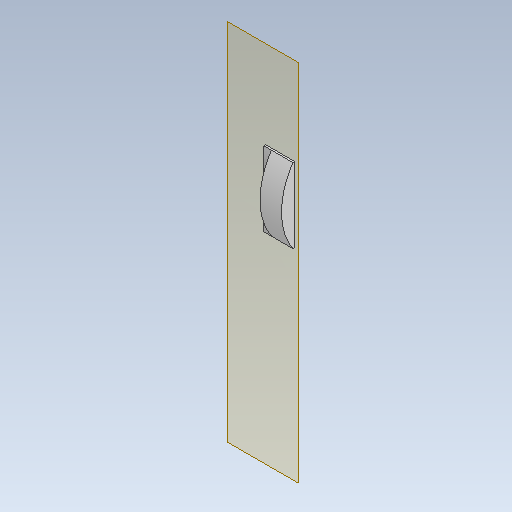
# Autodesk Inventor part: pully cover
Saved by Autodesk Inventor 2020 (Build 240168000, 168)
## iProperties
Created: 2020-03-07
Part Number: pully cover
Material: Generic
Document SubType Name: Modeling
Designer: jackm
Density: 1 g/cm^3
Appearance: Default
Author: jackm
Autodesk Inventor part; units mm, degrees
ref_plane "YZ Plane" through (0, 0, 0) normal (1, 0, 0) x (0, 1, 0)
ref_plane "XZ Plane" through (0, 0, 0) normal (0, 1, 0) x (-1, 0, 0)
ref_plane "XY Plane" through (0, 0, 0) normal (0, 0, 1) x (1, 0, 0)
ref_plane "Work Plane1" through (0, 0, 0) normal (0, 0, 1) x (1, 0, 0)
sketch "Sketch1" plane through (0, 0, 0) normal (0, 0, 1) x (1, 0, 0)
  line L0 (18.4366, 123.794) -> (43.8366, 123.794) construction
  line L1 (18.4366, 32.354) -> (18.4366, 123.794) construction
  line L2 (43.8366, 32.354) -> (18.4366, 32.354) construction
  circle A0 centre (9.9557, 104.744) radius 1.7 construction
  circle A1 centre (9.9557, 51.404) radius 1.7 construction
  line L3 (38.8366, 123.794) -> (18.4366, 123.794)
  line L4 (18.4366, 32.354) -> (38.8366, 32.354)
  circle A2 centre (9.9557, 104.744) radius 1.7
  circle A3 centre (9.9557, 51.404) radius 1.7
  line L5 (4.1111, 104.744) -> (4.1111, 123.794)
  line L6 (4.1111, 104.744) -> (4.1111, 32.354)
  line L7 (38.8366, 225.425) -> (38.8366, -225.425) construction
  line L8 (38.8366, 123.794) -> (38.8366, 32.354)
  line L9 (18.4366, 123.794) -> (18.4366, 32.354)
  line L10 (4.1111, 123.794) -> (4.1111, 128.794)
  line L11 (4.1111, 128.794) -> (43.8366, 128.794)
  line L12 (43.8366, 128.794) -> (43.8366, 32.354)
  line L13 (43.8366, 32.354) -> (43.8366, 27.354)
  line L14 (43.8366, 27.354) -> (4.1111, 27.354)
  line L15 (4.1111, 27.354) -> (4.1111, 32.354)
  point P0 (0, 0)
  dimension "d0" = 3.4
  dimension "d1" = 3.4
  dimension "d2" = 5
  dimension "d3" = 5
  constraints: 24 end point, 6 point on line, 4 perpendicular, 3 collinear, 2 centre point, 2 coincident, 1 parallel, 1 vertical
  measures "d0" diameter of A2
  measures "d1" diameter of A3
  measures "d2" distance of L5.end L10.end
  measures "d3" distance of L2.start L13.end
extrude "Extrusion1" add sketch "Sketch1" along normal blind 2.54
sketch "Sketch2" plane through (38.8366, 32.354, 0) normal (-1, 0, 0) x (0, 0, 1)
  line L0 (2.54, 91.44) -> (2.54, 0) projected
  line L1 (0, 91.44) -> (2.54, 91.44) projected
  arc A0 (2.54, 0) -> (2.54, 91.44) centre (-81.7195, 45.72) ccw
  line L2 (2.54, 96.44) -> (2.54, -5) projected
  arc A1 (2.54, -5) -> (2.54, 96.44) centre (-72.6611, 45.72) ccw
  point P0 (0, -32.354)
  constraints: 4 point on circle, 2 centre point
extrude "Extrusion2" add sketch "Sketch2" along normal up to surface (20.4 mm away) contours L2 A1 A0
sketch "Sketch3" plane through (38.8366, 32.354, 0) normal (1, 0, 0) x (0, 0, -1)
  arc A0 (-2.54, 96.44) -> (-2.54, -5) centre (72.6611, 45.72) ccw projected
  line L0 (-2.54, 96.44) -> (-2.54, -5)
  arc A1 (-2.54, 96.44) -> (-2.54, -5) centre (72.6611, 45.72) ccw
  point P0 (0, -32.354)
  constraints: 3 point on circle, 2 end point, 1 centre point, 1 concentric, 1 vertical
extrude "Extrusion3" add sketch "Sketch3" along normal up to surface (5 mm away)
sketch "Sketch4" plane through (18.4366, 78.074, -72.6611) normal (-1, 0, 0) x (0, 0, 1)
  arc A0 (75.2011, -50.72) -> (75.2011, 50.72) centre (0, 0) ccw projected
  line L0 (75.2011, 50.72) -> (75.2011, -50.72)
  arc A1 (75.2011, -50.72) -> (75.2011, 50.72) centre (0, 0) ccw
  point P0 (72.6611, -78.074)
  constraints: 2 end point, 2 point on circle, 1 centre point, 1 concentric, 1 vertical
extrude "Extrusion4" add sketch "Sketch4" along normal blind 3.81
body "Solid1"
